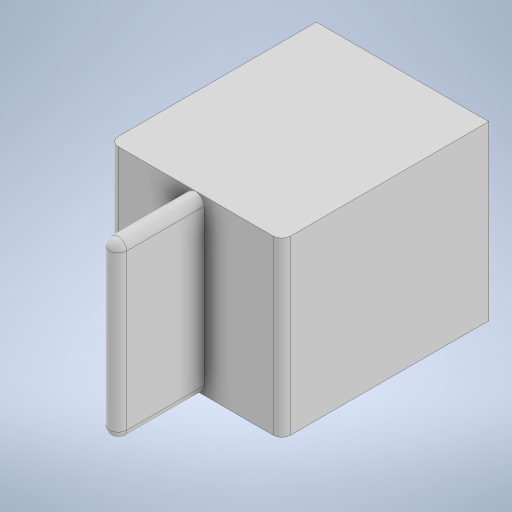
# Autodesk Inventor part: veg_kapcs_erzekelo_meretezett
Saved by Autodesk Inventor 2024 (Build 280153000, 153)
## iProperties
Created: 2024-03-06
Part Number: veg_kapcs_erzekelo_meretezett
Material: Generic
Document SubType Name: Modeling
Designer: Panka
Density: 1 g/cm^3
Appearance: Default
Author: Panka
Autodesk Inventor part; units mm, degrees
ref_plane "YZ Plane" through (0, 0, 0) normal (1, 0, 0) x (0, 1, 0)
ref_plane "XZ Plane" through (0, 0, 0) normal (0, 1, 0) x (-1, 0, 0)
ref_plane "XY Plane" through (0, 0, 0) normal (0, 0, 1) x (1, 0, 0)
sketch "Sketch1" plane through (0, 0, 0) normal (0, 1, 0) x (-1, 0, 0)
  line L0 (0, 0) -> (-20, 0)
  line L1 (-20, 0) -> (-20, -24)
  line L2 (-20, -24) -> (0, -24)
  line L3 (0, -24) -> (0, 0)
  line L4 (-9, 0) -> (-11, 0)
  line L5 (-11, 0) -> (-11, 10)
  line L6 (-11, 10) -> (-9, 10)
  line L7 (-9, 10) -> (-9, 0)
  dimension "d0" = 20
  dimension "d1" = 24
  dimension "d2" = 2
  dimension "d3" = 10
  dimension "d4" = 9
  constraints: 16 end point, 4 parallel, 2 horizontal, 2 perpendicular, 1 point on line
  measures "d0" distance of L2.end L1.end
  measures "d1" distance of L1.end L0.end
  measures "d2" distance of L5.end L6.end
  measures "d3" distance of L4.end L5.end
  measures "d4" distance of L4.start L0.start
extrude "Extrusion1" add sketch "Sketch1" along normal blind 20
fillet "Fillet1" radius 1 4 edges at (9, 20, 5) (9, 0, 5) (11, 0, 5) (11, 20, 5)
fillet "Fillet2" radius 1 4 edges at (11, 10, 10) (9.2927, 19.7073, 10) (9, 10, 10) (9.2927, 0.2927, 10)
fillet "Fillet3" radius 1 2 edges at (20, 10, 0) (0, 10, 0)
body "Solid1"
